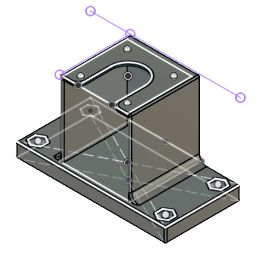
stepper_mount (Autodesk Fusion 360 design; units mm, degrees)
Autodesk Fusion 360 part; units mm, degrees
sketch "Sketch1" plane through (0, 0, 0) normal (0, 0, 1) x (1, 0, 0)
  line L0 (-50, 25) -> (50, 25)
  line L1 (50, 25) -> (50, -25)
  line L2 (50, -25) -> (-50, -25)
  line L3 (-50, -25) -> (-50, 25)
  line L4 (-50, 25) -> (50, -25) construction
  line L5 (50, 25) -> (-50, -25) construction
  dimension "d70" = 100
  dimension "d71" = 50
  constraint horizontal L0
  constraint perpendicular L0 L1
  constraint parallel L0 L2
  constraint parallel L1 L3
  constraint coincident L4 origin
  constraint coincident L5 origin
  measures "d70" distance of L1.end L2.end
  measures "d71" distance of L0.end L1.end
extrude "Extrude9" add sketch "Sketch1" along normal blind 10
sketch "Sketch7" plane through (0, 0, 10) normal (0, 0, 1) x (-1, 0, 0)
  line L0 (50, 25) -> (-50, 25)
  line L1 (-50, 25) -> (-50, -25)
  line L2 (-50, -25) -> (50, -25)
  line L3 (50, -25) -> (50, 25)
  line L4 (50, -25) -> (-50, -25)
  line L5 (-50, -25) -> (-50, 25)
  line L6 (-50, 25) -> (50, 25)
  line L7 (50, 25) -> (50, -25)
  line L8 (50, -25) -> (-50, 25) construction
  line L9 (-50, -25) -> (50, 25) construction
  line L10 (38.3, -19.9249) -> (42.5, -22.3497)
  line L11 (42.5, -22.3497) -> (46.7, -19.9249)
  line L12 (46.7, -19.9249) -> (46.7, -15.0751)
  line L13 (46.7, -15.0751) -> (42.5, -12.6503)
  line L14 (42.5, -12.6503) -> (38.3, -15.0751)
  line L15 (38.3, -15.0751) -> (38.3, -19.9249)
  line L16 (-46.7, -19.9249) -> (-42.5, -22.3497)
  line L17 (-42.5, -22.3497) -> (-38.3, -19.9249)
  line L18 (-46.7, -15.0751) -> (-46.7, -19.9249)
  line L19 (-42.5, -12.6503) -> (-46.7, -15.0751)
  line L20 (-38.3, -15.0751) -> (-42.5, -12.6503)
  line L21 (-38.3, -19.9249) -> (-38.3, -15.0751)
  line L22 (38.3, 15.0751) -> (42.5, 12.6503)
  line L23 (42.5, 12.6503) -> (46.7, 15.0751)
  line L24 (38.3, 19.9249) -> (38.3, 15.0751)
  line L25 (42.5, 22.3497) -> (38.3, 19.9249)
  line L26 (46.7, 19.9249) -> (42.5, 22.3497)
  line L27 (46.7, 15.0751) -> (46.7, 19.9249)
  line L28 (-46.7, 15.0751) -> (-42.5, 12.6503)
  line L29 (-42.5, 12.6503) -> (-38.3, 15.0751)
  line L30 (-46.7, 19.9249) -> (-46.7, 15.0751)
  line L31 (-42.5, 22.3497) -> (-46.7, 19.9249)
  line L32 (-38.3, 19.9249) -> (-42.5, 22.3497)
  line L33 (-38.3, 15.0751) -> (-38.3, 19.9249)
  line L34 (-23.5, -25) -> (23.5, -25)
  line L35 (23.5, -25) -> (23.5, 22)
  line L36 (23.5, 22) -> (-23.5, 22)
  line L37 (-23.5, 22) -> (-23.5, -25)
  point P0 (42.5, -17.5)
  point P1 (42.5, -17.5)
  point P2 (-42.5, -17.5)
  point P3 (42.5, 17.5)
  point P4 (-42.5, 17.5)
  point P5 (0, -25)
  dimension "d82" = 100
  dimension "d83" = 50
  dimension "d84" = 7.5
  dimension "d85" = 7.5
  dimension "d90" = 4.2
  dimension "d93" = -85
  dimension "d94" = 35
  dimension "d102" = 47
  dimension "d103" = 47
  dimension "d104" = 26.5
  constraint horizontal L4
  constraint perpendicular L4 L5
  constraint parallel L4 L6
  constraint parallel L5 L7
  constraint coincident L8 origin
  constraint coincident L9 origin
  constraint coincident P1 P0
  constraint midpoint L4 P5
  constraint horizontal L34
  constraint vertical L35
  constraint horizontal L36
  constraint vertical L37
  constraint coincident L2 L34.start
  measures "d82" distance of L0.end L0.start
  measures "d83" distance of L1.end L0.end
  measures "d84" distance of L7 P1
  measures "d85" distance of L4 P1
  measures "d90" distance of P1 L15
  measures "d102" distance of L34.start L34.end
  measures "d103" distance of L34.start L36.end
  measures "d104" distance of L5 L37
hole "Hole2" at (-42.5, 17.5, 10) at (42.5, 17.5, 10) at (42.5, -17.5, 10) at (-42.5, -17.5, 10) direction (0, 0, -1) diameter 5.2 depth 10 tip angle 180
extrude "Extrude10" cut sketch "Sketch7" against normal blind 5 contours L10 L11 L12 L13 L14 L15 | L16 L17 L18 L19 L20 L21 | L22 L23 L24 L25 L26 L27 | L28 L29 L30 L31 L32 L33
extrude "Extrude11" add sketch "Sketch7" along normal blind 50 contours L2 L4 L34 L35 L36 L37
sketch "Sketch8" plane through (0, -22, 0) normal (0, -1, 0) x (1, 0, 0)
  line L0 (-23.5, 10) -> (23.5, 10)
  line L1 (23.5, 10) -> (23.5, 60)
  line L2 (23.5, 60) -> (-23.5, 60)
  line L3 (-23.5, 60) -> (-23.5, 10)
  line L4 (-21.5, 58) -> (21.5, 58)
  line L5 (21.5, 58) -> (21.5, 10)
  line L6 (21.5, 10) -> (-21.5, 10)
  line L7 (-21.5, 10) -> (-21.5, 58)
  dimension "d107" = 43
  dimension "d108" = 48
  dimension "d109" = 2
  dimension "d110" = 2
  constraint horizontal L4
  constraint vertical L5
  constraint horizontal L6
  constraint vertical L7
  measures "d107" distance of L4.start L4.end
  measures "d108" distance of L4.start L6.end
  measures "d109" distance of L3 L7
  measures "d110" distance of L2 L4
extrude "Extrude12" cut sketch "Sketch8" against normal blind 43 contours L0 L4 L5 L6 L7
sketch "Sketch9" plane through (0, 0, 60) normal (0, 0, 1) x (-1, 0, 0)
  line L0 (-23.5, 22) -> (-23.5, -25)
  line L1 (-23.5, -25) -> (23.5, -25)
  line L2 (23.5, -25) -> (23.5, 22)
  line L3 (23.5, 22) -> (-23.5, 22)
  line L4 (-11.2, 0) -> (-11.2, 22)
  line L5 (11.2, 0) -> (11.2, 22)
  arc A0 (-11.2, 0) -> (11.2, 0) centre (0, 0) ccw
  line L6 (21.5, -21) -> (-21.5, -21)
  line L7 (-21.5, -21) -> (-21.5, 22)
  line L8 (-21.5, 22) -> (21.5, 22)
  line L9 (21.5, 22) -> (21.5, -21)
  line L10 (23.5, -25) -> (23.5, 22)
  line L11 (50, -25) -> (-50, -25)
  point P0 (15.5, -15)
  point P1 (-15.5, -15)
  point P2 (15.5, 16)
  point P3 (-15.5, 16)
  dimension "d113" = 22.4
  dimension "d118" = -31
  dimension "d119" = 31
  dimension "d120" = 43
  dimension "d121" = 43
  dimension "d122" = 2
  dimension "d123" = 4
  dimension "d124" = 6
  dimension "d125" = 6
  constraint coincident A0.centre origin
  constraint coincident L3 L4.end
  constraint tangent L4 A0
  constraint perpendicular L3 L4
  constraint coincident L3 L5.end
  constraint tangent L5 A0
  constraint perpendicular L3 L5
  constraint horizontal L6
  constraint vertical L7
  constraint horizontal L8
  constraint vertical L9
  measures "d113" diameter of A0
  measures "d120" distance of L6.start L6.end
  measures "d121" distance of L6.start L8.end
  measures "d122" distance of L9 L10
  measures "d123" distance of L6 L11
  measures "d124" distance of P0 L6
  measures "d125" distance of P0 L9
extrude "Extrude13" cut sketch "Sketch9" against normal blind 2 contours L3 L4 L5 A0 L8
hole "Hole3" at (-15.5, 15, 60) at (15.5, 15, 60) at (15.5, -16, 60) at (-15.5, -16, 60) direction (0, 0, -1) diameter 3.4 depth 2 tip angle 180
fillet "Fillet13" radius 5 2 edges at (-11.2, -22, 59) (11.2, -22, 59)
fillet "Fillet13" radius 1 47 edges at (0, -25, 10) (0, -25, 0) (50, -25, 5) (50, 0, 10) (50, 0, 0) (50, 25, 5) (36.75, 25, 10) (0, 25, 0) (-36.75, 25, 10) (-50, 25, 5) (-50, 0, 10) (-50, 0, 0) (-50, -25, 5) (-23.5, 25, 35) (23.5, 25, 35) (0, 25, 60) (38.3, 17.5, 10) (40.4, 21.1373, 10) (44.6, 21.1373, 10) (46.7, 17.5, 10) (44.6, 13.8627, 10) (40.4, 13.8627, 10) (40.4, -13.8627, 10) (44.6, -13.8627, 10) (38.3, -17.5, 10) (40.4, -21.1373, 10) (44.6, -21.1373, 10) (46.7, -17.5, 10) (-38.3, 17.5, 10) (-40.4, 21.1373, 10) (-44.6, 21.1373, 10) (-46.7, 17.5, 10) (-44.6, 13.8627, 10) (-40.4, 13.8627, 10) (-40.4, -13.8627, 10) (-44.6, -13.8627, 10) (-46.7, -17.5, 10) (-44.6, -21.1373, 10) (-40.4, -21.1373, 10) (-38.3, -17.5, 10) (-11.2, -11, 60) (0, 11.2, 60) (11.2, -11, 60) (-17.35, -22, 60) (-23.5, -22, 35) (17.35, -22, 60) (23.5, -22, 35)
fillet "Fillet13" radius 1 2 edges at (21.5, -22, 34) (-21.5, -22, 34)
fillet "Fillet13" radius 1 2 edges at (-23.5, 1.5, 60) (23.5, 1.5, 60)
fillet "Fillet13" radius 5 2 edges at (23.5, 1.5, 10) (-23.5, 1.5, 10)
